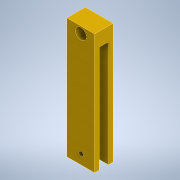
# Autodesk Inventor part: pendel
Saved by Autodesk Inventor 2021 (Build 250183000, 183)
## iProperties
Created: 2021-02-09
Part Number: pendel
Material: Generic
Document SubType Name: Modeling
Designer: Emil
Density: 1 g/cm^3
Appearance: Gold
Author: Emil
Autodesk Inventor part; units mm, degrees
ref_plane "YZ Plane" through (0, 0, 0) normal (1, 0, 0) x (0, 1, 0)
sketch "Sketch1" plane through (0, 0, 0) normal (0, 0, 1) x (1, 0, 0)
  point P0 (0, 0)
sketch "Sketch2" plane through (0, 0, 0) normal (0, 0, 1) x (1, 0, 0)
  line L0 (-15, 130) -> (15, 130)
  line L1 (15, 130) -> (15, 0)
  line L2 (15, 0) -> (-15, 0)
  line L3 (-15, 0) -> (-15, 130)
  point P0 (0, 0)
  point P1 (0, 0)
  dimension "d0" = 30
  dimension "d1" = 130
  constraints: 8 end point, 2 parallel, 1 coincident, 1 horizontal, 1 midpoint, 1 perpendicular
  measures "d0" distance of L0.start L0.end
  measures "d1" distance of L0.end L1.end
extrude "Extrusion1" add sketch "Sketch2" along normal blind 5
ref_plane "Work Plane1" through (0, 0, -10) normal (0, 0, -1) x (-1, 0, 0)
sketch "Sketch4" plane through (0, 0, -10) normal (0, 0, -1) x (-1, 0, 0)
  line L0 (-15, 0) -> (-15, 130) projected
  line L1 (15, 0) -> (-15, 0) projected
  line L2 (-15, 130) -> (15, 130)
  line L3 (15, 130) -> (15, 0)
  line L4 (15, 0) -> (-15, 0)
  line L5 (-15, 0) -> (-15, 130)
  point P0 (0, 0)
  constraints: 8 end point, 2 parallel, 1 horizontal, 1 perpendicular
extrude "Extrusion3" add sketch "Sketch4" along normal blind 5
sketch "Sketch5" plane through (0, 0, -10) normal (0, 0, 1) x (1, 0, 0)
  line L0 (-15, 130) -> (-15, 0) projected
  line L1 (15, 130) -> (15, 0) projected
  line L2 (-15, 130) -> (15, 130)
  line L3 (15, 130) -> (15, 115)
  line L4 (15, 115) -> (-15, 115)
  line L5 (-15, 115) -> (-15, 130)
  point P0 (0, 0)
  point P1 (15, 130)
  dimension "d12" = 15
  constraints: 8 end point, 2 parallel, 1 horizontal, 1 perpendicular, 1 point on line
  measures "d12" distance between parallel lines of L4 L2
extrude "Extrusion4" add sketch "Sketch5" along normal blind 10
sketch "Sketch6" plane through (0, 0, -10) normal (0, 0, 1) x (1, 0, 0)
  circle A0 centre (0, 10) radius 2.5
  line L0 (-15, 0) -> (15, 0) projected
  point P0 (0, 0)
  dimension "d15" = 5
  dimension "d16" = 10
  dimension "d45" = 18.0278
  constraints: 1 centre point
  measures "d15" diameter of A0
  measures "d16" distance from line of L0 A0.centre
  measures "d45" distance of L0.end A0.centre
extrude "Extrusion5" cut sketch "Sketch6" along normal blind 15 and the other way blind 5
ref_plane "Work Plane2" through (0, 0, -5) normal (0, 0, 1) x (1, 0, 0)
sketch "Sketch9" plane through (0, 0, 5) normal (0, 0, 1) x (1, 0, 0)
  line L0 (15, 130) -> (-15, 130) projected
  line L1 (15, 0) -> (15, 130) projected
  line L2 (0, 84.3715) -> (0, -83.7026)
  line L3 (-15, 0) -> (15, 0) projected
  line L4 (-15, 122.5) -> (15, 122.5)
  line L5 (-15, 115) -> (15, 115) projected
  circle A0 centre (0, 122.5) radius 6
  point P0 (0, 0)
  point P1 (0, 0)
  dimension "d41" = 7.5
  dimension "d42" = 12
  dimension "d46" = 15
  dimension "d47" = 45.6285
  dimension "d48" = 213.7026
  constraints: 4 end point, 2 midpoint, 2 point on line, 1 centre point, 1 perpendicular, 1 vertical
  measures "d41" distance between parallel lines of L5 L4
  measures "d42" diameter of A0
  measures "d46" distance from line of A0.centre L1
  measures "d47" distance from line of L2.start L0
  measures "d48" distance from line of L2.end L0
extrude "Extrusion7" cut sketch "Sketch9" against normal blind 20
body "Solid1"
